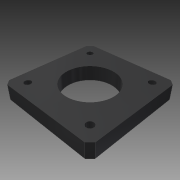
# Autodesk Inventor part: x_motor_spacer
Saved by Autodesk Inventor 2014 (Build 180170000, 170)
## iProperties
Created: 2013-11-07
Part Number: x_motor_spacer
Material: Plywood, Finish
Document SubType Name: Modeling
Designer: buben
Density: 0.552 g/cm^3
Appearance: Plywood - New
Author: buben
Subject: Laser Cutted
Autodesk Inventor part; units mm, degrees
ref_plane "YZ Plane" through (0, 0, 0) normal (1, 0, 0) x (0, 1, 0)
ref_plane "XZ Plane" through (0, 0, 0) normal (0, 1, 0) x (-1, 0, 0)
ref_plane "XY Plane" through (0, 0, 0) normal (0, 0, 1) x (1, 0, 0)
sketch "Sketch1" plane through (0, 0, 0) normal (0, 0, 1) x (1, 0, 0)
  line L0 (2, 0) -> (40.67, 0)
  line L1 (42.67, 2) -> (42.67, 40.67)
  line L2 (40.67, 42.67) -> (2, 42.67)
  line L3 (0, 40.67) -> (0, 2)
  line L4 (2, 42.67) -> (0, 40.67)
  line L5 (0, 2) -> (2, 0)
  line L6 (40.67, 0) -> (42.67, 2)
  line L7 (42.67, 40.67) -> (40.67, 42.67)
  circle A0 centre (21.335, 21.335) radius 11.5
  line L8 (5.835, 36.835) -> (36.835, 36.835) construction
  line L9 (36.835, 36.835) -> (36.835, 5.835) construction
  line L10 (36.835, 5.835) -> (5.835, 5.835) construction
  line L11 (5.835, 5.835) -> (5.835, 36.835) construction
  circle A1 centre (5.835, 36.835) radius 1.6
  circle A2 centre (36.835, 36.835) radius 1.6
  circle A3 centre (36.835, 5.835) radius 1.6
  circle A4 centre (5.835, 5.835) radius 1.6
  point P0 (0, 0)
  point P1 (42.67, 42.67)
  point P2 (42.67, 0)
  point P3 (0, 42.67)
  point P4 (42.67, 21.335)
  point P5 (21.335, 42.67)
  point P6 (21.335, 36.835)
  point P7 (36.835, 21.335)
  dimension "d0" = 2
  dimension "d1" = 2
  dimension "d2" = 2
  dimension "d3" = 2
  dimension "d4" = 2
  dimension "d5" = 2
  dimension "d6" = 2
  dimension "d7" = 2
  dimension "d8" = 42.67
  dimension "d9" = 42.67
  dimension "d10" = 23
  dimension "d11" = 31
  dimension "d12" = 31
  dimension "d13" = 3.2
  dimension "d14" = 3.2
  dimension "d15" = 3.2
  dimension "d16" = 3.2
  constraints: 24 end point, 8 point on line, 5 centre point, 4 coincident, 4 midpoint, 4 parallel, 2 horizontal, 2 horizontal alignment, 2 perpendicular, 2 vertical alignment
  measures "d0" distance of L2.end point (0, 42.67)
  measures "d1" distance of L3.start point (0, 42.67)
  measures "d2" distance of L3.end point (0, 0)
  measures "d3" distance of L0.start point (0, 0)
  measures "d4" distance of L0.end point (42.67, 0)
  measures "d5" distance of L1.start point (42.67, 0)
  measures "d6" distance of L1.end point (42.67, 42.67)
  measures "d7" distance of L2.start point (42.67, 42.67)
  measures "d8" distance between parallel lines of L1 L3
  measures "d9" distance between parallel lines of L2 L0
  measures "d10" diameter of A0
  measures "d11" distance of L8.start L8.end
  measures "d12" distance of L8.end L9.end
  measures "d13" diameter of A4
  measures "d14" diameter of A3
  measures "d15" diameter of A1
  measures "d16" diameter of A2
extrude "Extrusion1" add sketch "Sketch1" along normal blind 6.5
equation "\"d1\" = d0"
equation "\"d2\" = d0"
equation "\"d3\" = d2"
equation "\"d4\" = d0"
equation "\"d5\" = d4"
equation "\"d6\" = d0"
equation "\"d7\" = d6"
body "Solid1"
